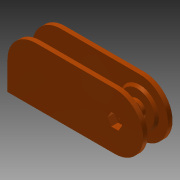
# Autodesk Inventor part: z pulley holder
Saved by Autodesk Inventor 2014 (Build 180170000, 170)
## iProperties
Created: 2013-07-26
Part Number: z pulley holder
Material: Generic
Document SubType Name: Modeling
Designer: employee
Density: 1 g/cm^3
Mass: 6.87177 g
Surface Area: 68.4002 cm^2
Volume: 6.87177 cm^3
Appearance: Smooth - Light Orange
Author: employee
Autodesk Inventor part; units mm, degrees
ref_plane "YZ Plane" through (0, 0, 0) normal (1, 0, 0) x (0, 1, 0)
ref_plane "XZ Plane" through (0, 0, 0) normal (0, 1, 0) x (-1, 0, 0)
ref_plane "XY Plane" through (0, 0, 0) normal (0, 0, 1) x (1, 0, 0)
sketch "Sketch1" plane through (0, 0, 0) normal (0, 0, 1) x (1, 0, 0)
  line L0 (-25, 6.5) -> (0, 6.5)
  line L1 (0, 6.5) -> (0, -6.5)
  line L2 (0, -6.5) -> (-25, -6.5)
  line L3 (-25, -6.5) -> (-25, 6.5)
  point P0 (0, 0)
  point P1 (0, 0)
  dimension "d0" = 13
  dimension "d2" = 25
  constraints: 8 end point, 2 coincident, 2 parallel, 1 horizontal, 1 midpoint, 1 perpendicular
  measures "d0" distance of L2.end L0.start
  measures "d2" distance of L1.end L2.end
extrude "Extrusion1" add sketch "Sketch1" along normal blind 5
sketch "Sketch2" plane through (-25, -6.5, 0) normal (0, -1, 0) x (1, 0, 0)
  line L0 (25, 0) -> (25, 5) projected
  line L1 (0, 0) -> (60, 0)
  line L2 (60, 0) -> (60, 25)
  line L3 (60, 25) -> (0, 25)
  line L4 (0, 25) -> (0, 0)
  dimension "d5" = 35
  dimension "d6" = 25
  constraints: 8 end point, 2 parallel, 1 horizontal, 1 perpendicular
  measures "d5" distance between parallel lines of L2 L0
  measures "d6" distance of L1.end L2.end
extrude "Extrusion2" add sketch "Sketch2" against normal blind 2
fillet "Fillet1" radius 12.5 3 edges at (35, -5.5, 0) (35, -5.5, 25) (-25, -5.5, 25)
sketch "Sketch4" plane through (-25, -4.5, 0) normal (0, 1, 0) x (1, 0, 0)
  arc A0 (47.5, -25) -> (47.5, 0) centre (47.5, -12.5) ccw projected
  circle A1 centre (47.5, -12.5) radius 7.5
  dimension "d10" = 15
  constraints: 1 centre point, 1 coincident
  measures "d10" diameter of A1
extrude "Extrusion3" add sketch "Sketch4" along normal blind 1
chamfer "Chamfer1" distance 1 angle 45 1 edges at (15, -4.5, 12.5)
sketch "Sketch5" plane through (22.5, -3.5, 12.5) normal (0, 1, 0) x (1, 0, 0)
  circle A0 centre (0, 0) radius 7.5 projected
  circle A1 centre (0, 0) radius 3.75
  point P0 (-22.5, 12.5)
  dimension "d17" = 7.5
  constraints: 1 centre point, 1 coincident
  measures "d17" diameter of A1
extrude "Extrusion4" add sketch "Sketch5" along normal blind 1.5 contours A1
sketch "Sketch6" plane through (0, 6.5, 5) normal (1, 0, 0) x (0, 0, -1)
  line L0 (-3.75, -8.5) -> (-11.25, -8.5) projected
  line L1 (-11.25, -10) -> (-3.75, -10) projected
  line L2 (-3.75, -10) -> (-5.25, -8.5)
  line L3 (-3.75, -8.5) -> (-3.75, -10)
  line L4 (-3.75, -8.5) -> (-5.25, -8.5)
  point P0 (5, -6.5)
  constraints: 6 end point, 3 perpendicular, 1 point on line
extrude "Extrusion5" cut sketch "Sketch6" along normal through all
mirror "Mirror1" about plane through (0, 0, 0) normal (0, 1, 0) of "Extrusion4", "Extrusion3", "Chamfer1", "Fillet1", "Extrusion2", "Extrusion5"
sketch "Sketch7" plane through (0, 0, 5) normal (0, 0, 1) x (1, 0, 0)
  line L0 (-25, 4.5) -> (-25, -4.5) projected
  line L1 (0, -4.5) -> (0, 4.5) projected
  line L2 (-25, 0) -> (0, 0)
  circle A0 centre (-20, 0) radius 1.55
  circle A1 centre (-5, 0) radius 1.55
  dimension "d23" = 5
  dimension "d24" = 5
  dimension "d25" = 3.1
  constraints: 2 centre point, 2 end point, 2 point on line, 1 equal radius, 1 midpoint, 1 perpendicular
  measures "d23" distance of L2.end A1.centre
  measures "d24" distance from line of L0 A0.centre
  measures "d25" diameter of A1
extrude "Extrusion6" cut sketch "Sketch7" against normal through all
sketch "Sketch8" plane through (0, 0, 5) normal (0, 0, 1) x (1, 0, 0)
  circle A0 centre (-5, 0) radius 1.55 projected
  circle A1 centre (-20, 0) radius 1.55 projected
  line L0 (-16.7668, 0) -> (-18.3834, -2.8)
  line L1 (-18.3834, -2.8) -> (-21.6166, -2.8)
  line L2 (-21.6166, -2.8) -> (-23.2332, 0)
  line L3 (-23.2332, 0) -> (-21.6166, 2.8)
  line L4 (-21.6166, 2.8) -> (-18.3834, 2.8)
  line L5 (-18.3834, 2.8) -> (-16.7668, 0)
  line L6 (-8.2332, 0) -> (-6.6166, 2.8)
  line L7 (-6.6166, 2.8) -> (-3.3834, 2.8)
  line L8 (-3.3834, 2.8) -> (-1.7668, 0)
  line L9 (-1.7668, 0) -> (-3.3834, -2.8)
  line L10 (-3.3834, -2.8) -> (-6.6166, -2.8)
  line L11 (-6.6166, -2.8) -> (-8.2332, 0)
  point P0 (0, 0)
  dimension "d28" = 5.6
  constraints: 24 end point, 2 coincident, 2 horizontal, 1 collinear, 26 other
  measures "d28" distance between parallel lines of L10 L7
extrude "Extrusion7" cut sketch "Sketch8" against normal blind 2.5
sketch "Sketch9" plane through (-12.5, 6.5, 25) normal (0, 1, 0) x (1, 0, 0)
  arc A0 (35, 0) -> (35, 25) centre (35, 12.5) ccw projected
  circle A1 centre (35, 12.5) radius 1.6
  point P0 (12.5, 25)
  dimension "d32" = 3.2
  constraints: 1 centre point, 1 coincident
  measures "d32" diameter of A1
extrude "Extrusion8" cut sketch "Sketch9" against normal through all
sketch "Sketch10" plane through (-12.5, 6.5, 25) normal (0, 1, 0) x (1, 0, 0)
  circle A0 centre (35, 12.5) radius 1.6 projected
  arc A1 (35, 0) -> (35, 25) centre (35, 12.5) ccw projected
  circle A2 centre (35, 12.5) radius 3.25
  point P0 (12.5, 25)
  dimension "d36" = 6.5
  constraints: 1 centre point, 1 coincident
  measures "d36" diameter of A2
extrude "Extrusion9" cut sketch "Sketch10" against normal blind 3
sketch "Sketch11" plane through (-12.5, -6.5, 25) normal (0, -1, 0) x (1, 0, 0)
  circle A0 centre (35, -12.5) radius 1.6 projected
  arc A1 (35, -25) -> (35, 0) centre (35, -12.5) ccw projected
  line L0 (31.7668, -12.5) -> (33.3834, -9.7)
  line L1 (33.3834, -9.7) -> (36.6166, -9.7)
  line L2 (36.6166, -9.7) -> (38.2332, -12.5)
  line L3 (38.2332, -12.5) -> (36.6166, -15.3)
  line L4 (36.6166, -15.3) -> (33.3834, -15.3)
  line L5 (33.3834, -15.3) -> (31.7668, -12.5)
  point P0 (12.5, -25)
  point P1 (35, -9.7)
  dimension "d40" = 5.6
  constraints: 12 end point, 1 coincident, 1 horizontal alignment, 1 midpoint, 13 other
  measures "d40" vertical distance of L3.end point (35, -9.7)
extrude "Extrusion10" cut sketch "Sketch11" against normal blind 3
body "Solid1"
